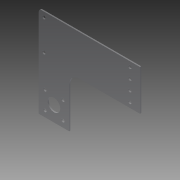
# Autodesk Inventor part: Lexan flexible Arm Mount
Saved by Autodesk Inventor 2014 (Build 180170000, 170)
## iProperties
Created: 2014-02-11
Part Number: Lexan flexible Arm Mount
Material: Polycarbonate, Clear
Document SubType Name: Modeling
Designer: Michael
Density: 1.2 g/cm^3
Appearance: Polycarbonate - Clear
Author: Michael
Autodesk Inventor part; units mm, degrees
ref_plane "YZ Plane" through (0, 0, 0) normal (1, 0, 0) x (0, 1, 0)
ref_plane "XZ Plane" through (0, 0, 0) normal (0, 1, 0) x (-1, 0, 0)
ref_plane "XY Plane" through (0, 0, 0) normal (0, 0, 1) x (1, 0, 0)
sketch "Sketch1" plane through (0, 0, 0) normal (0, 0, 1) x (1, 0, 0)
  line L0 (0, 0) -> (0, 111.125)
  line L1 (3.175, 114.3) -> (127, 114.3)
  line L2 (127, 63.5) -> (127, 114.3)
  line L3 (0, 0) -> (38.1, 0)
  line L4 (38.1, 0) -> (38.1, 50.8)
  line L5 (50.8, 63.5) -> (127, 63.5)
  circle A0 centre (19.05, 19.05) radius 7.9375
  line L6 (22.7162, 25.4) -> (26.3823, 19.05) construction
  line L7 (26.3823, 19.05) -> (22.7162, 12.7) construction
  line L8 (22.7162, 12.7) -> (15.3838, 12.7) construction
  line L9 (15.3838, 12.7) -> (11.7177, 19.05) construction
  line L10 (11.7177, 19.05) -> (15.3838, 25.4) construction
  line L11 (15.3838, 25.4) -> (22.7162, 25.4) construction
  arc A1 (50.8, 63.5) -> (38.1, 50.8) centre (50.8, 50.8) ccw
  arc A2 (3.175, 114.3) -> (0, 111.125) centre (3.175, 111.125) ccw
  circle A3 centre (114.3, 107.95) radius 2.0828
  circle A4 centre (114.3, 95.25) radius 2.0828
  circle A5 centre (114.3, 82.55) radius 2.0828
  circle A6 centre (114.3, 69.85) radius 2.0828
  circle A7 centre (7.8247, 7.8247) radius 2.0828
  line L12 (7.8247, 7.8247) -> (19.05, 19.05) construction
  circle A8 centre (30.2753, 7.8247) radius 2.0828
  circle A9 centre (30.2753, 30.2753) radius 2.0828
  circle A10 centre (7.8247, 30.2753) radius 2.0828
  circle A11 centre (6.35, 107.95) radius 2.0828
  circle A12 centre (6.35, 69.85) radius 2.0828
  point P0 (0, 114.3)
  point P1 (38.1, 63.5)
  dimension "d0" = 114.3
  dimension "d1" = 127
  dimension "d5" = 38.1
  dimension "d7" = 15.875
  dimension "d8" = 12.7
  dimension "d9" = 19.05
  dimension "d10" = 19.05
  dimension "d11" = 12.7
  dimension "d12" = 3.175
  dimension "d13" = 4.1656
  dimension "d14" = 12.7
  dimension "d15" = 6.35
  dimension "d18" = 12.7
  dimension "d23" = 4.1656
  dimension "d25" = 15.875
  dimension "d26" = 45
  dimension "d29" = 360
  dimension "d31" = 6.35
  dimension "d32" = 6.35
  dimension "d35" = 38.1
  dimension "d40" = 50.8
  constraints: 26 end point, 13 centre point, 5 perpendicular, 4 point on circle, 4 point on line, 4 tangent, 3 vertical, 1 coincident, 1 equal radius, 1 horizontal, 30 other
  measures "d0" distance of L0.start point (0, 114.3)
  measures "d1" distance of point (0, 114.3) L1.end
  measures "d5" distance of L0.start L3.end
  measures "d7" diameter of A0
  measures "d8" distance between parallel lines of L11 L8
  measures "d9" distance from line of A0.centre L0
  measures "d10" distance from line of L3 A0.centre
  measures "d11" radius of A1
  measures "d12" radius of A2
  measures "d13" diameter of A3
  measures "d14" distance from line of L2 A3.centre
  measures "d15" distance from line of L1 A3.centre
  measures "d18" distance of A3.centre A4.centre
  measures "d23" diameter of A7
  measures "d25" distance of L12.end L12.start
  measures "d26" angle of L8 L12
  measures "d31" distance from line of L1 A11.centre
  measures "d32" distance from line of L0 A11.centre
  measures "d35" distance of A11.centre A12.centre
  measures "d40" distance of L2.start L1.end
extrude "Extrusion1" add sketch "Sketch1" along normal blind 1.5875
body "Solid1"
